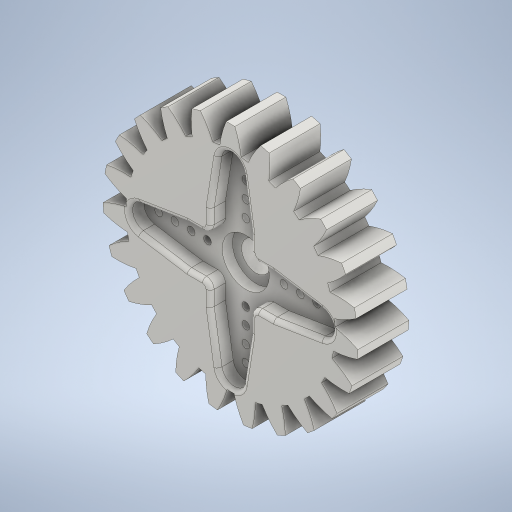
# Autodesk Inventor part: Engrenagem menor
Saved by Autodesk Inventor 2024.1 (Build 281209000, 209)
## iProperties
CustomPartVersion: 1
Created: 2024-11-07
Part Number: Engrenagem menor
Material: Steel
Document SubType Name: Modeling
Designer: dimit
Categories: <?xml version="1.0" encoding="UTF-16"?> <MemberInstance><Categories><FamilyTemplate><FamilyTemplateParameter ValueType="xs:double" Id="1" ObjectReferenceKey="da_z" ObjectType="kUserParameterObject"/><FamilyTemplateParameter ValueType="xs:double" Id="2" ObjectReferenceKey="da_b" ObjectType="kUserParameterObject"/><FamilyTemplateParameter ValueType="xs:double" Id="3" ObjectReferenceKey="da_beta" ObjectType="kUserParameterObject"/><FamilyTemplateParameter ValueType="xs:double" Id="4" ObjectReferenceKey="da_da" ObjectType="kUserParameterObject"/><FamilyTemplateParameter ValueType="xs:double" Id="5" ObjectReferenceKey="da_aw" ObjectType="kUserParameterObject"/><FamilyTemplateParameter ValueType="xs:string" Id="6" ObjectReferenceKey="EAIAABAAAACIAQAAAAAAAIAAAAAAAAAA" ObjectType="83910656" SubObjectId="SurfaceGeometry"/></FamilyTemplate><ParamToTemplateMap><ParamToTemplate CategoryParameter="//CategoryParameter[@InternalName='046C89C9-8512-4d59-83FE-43B91F4F132A']" TemplateParameter="1"/><ParamToTemplate CategoryParameter="//CategoryParameter[@InternalName='2552DF32-E462-4b46-AEBF-C6C7768E72AC']" TemplateParameter="2"/><ParamToTemplate CategoryParameter="//CategoryParameter[@InternalName='C9EE641D-15FC-4fae-A226-E94C4372FDD7']" TemplateParameter="3"/><ParamToTemplate><ParamToTemplate CategoryParameter="//CategoryParameter[@InternalName='00B6519A-459B-49c7-AD84-2E56D39A5744']" ConstantValue="0.000000"/></ParamToTemplate><ParamToTemplate><ParamToTemplate CategoryParameter="//CategoryParameter[@InternalName='04B31F0E-C7A6-4894-AA32-9629BEFACF47']" ConstantValue="1.000000"/></ParamToTemplate><ParamToTemplate><ParamToTemplate CategoryParameter="//CategoryParameter[@InternalName='43CBEC2E-7847-49e7-A936-2F7889FCB2D9']" ConstantValue="0.250000"/></ParamToTemplate><ParamToTemplate><ParamToTemplate CategoryParameter="//CategoryParameter[@InternalName='B1EFC894-105D-4ebd-86BF-FA20ED196853']" ConstantValue="0.333500"/></ParamToTemplate><ParamToTemplate><ParamToTemplate CategoryParameter="//CategoryParameter[@InternalName='51175063-3D10-4879-93E8-6246FE8B403D']" ConstantValue="2060000000.000000"/></ParamToTemplate><ParamToTemplate><ParamToTemplate CategoryParameter="//CategoryParameter[@InternalName='A3A52E27-4454-46a9-B0BD-C932399B70AF']" ConstantValue="0.300000"/></ParamToTemplate><ParamToTemplate><ParamToTemplate CategoryParameter="//CategoryParameter[@InternalName='91B76062-C214-41d9-B1B9-14D2AB99603D']" ConstantValue="0.200000"/></ParamToTemplate><ParamToTemplate><ParamToTemplate CategoryParameter="//CategoryParameter[@InternalName='374E806E-8B8A-4dda-A9AA-1039D6500AD2']" ConstantValue="5.000000"/></ParamToTemplate><ParamToTemplate><ParamToTemplate CategoryParameter="//CategoryParameter[@InternalName='2D373A89-B862-43d6-8D0B-0CBF12AB9F6C']" ConstantValue="0.349066"/></ParamToTemplate><ParamToTemplate CategoryParameter="//CategoryParameter[@InternalName='37777632-D6A2-4fac-9D53-DB8ACD95C989']" TemplateParameter="4"/><ParamToTemplate CategoryParameter="//CategoryParameter[@InternalName='FD1017F1-B727-4f7e-9707-0F86F1FF9423']" TemplateParameter="5"/><ParamToTemplate><ParamToTemplate CategoryParameter="//CategoryParameter[@InternalName='9E1B4470-B2D3-4ff1-B813-535BB4CDF51A']" ConstantValue="3520000.000000"/></ParamToTemplate><ParamToTemplate><ParamToTemplate CategoryParameter="//CategoryParameter[@InternalName='F8452263-BFF6-458c-9FB1-07C4B99E95CD']" ConstantValue="11400000.000000"/></ParamToTemplate><ParamToTemplate><ParamToTemplate CategoryParameter="//CategoryParameter[@InternalName='3E3BB259-FD49-497f-8171-6EBC954A3479']" ConstantValue="2.000000"/></ParamToTemplate><ParamToTemplate CategoryParameter="//CategoryParameter[@InternalName='27C3BAF2-7550-4e4b-AE2C-0DB134B7D9B7']" TemplateParameter="6"/></ParamToTemplateMap><Category DisplayName="Gear" InternalName="DC85795E-93AB-48d5-8EEE-5A27447B64BD" Mnemonic="Gear"><CategoryParameter DisplayName="z" InternalName="046C89C9-8512-4d59-83FE-43B91F4F132A" Mnemonic="z"/><CategoryParameter DisplayName="b" InternalName="2552DF32-E462-4b46-AEBF-C6C7768E72AC" Mnemonic="b"/><CategoryParameter DisplayName="||b|" InternalName="C9EE641D-15FC-4fae-A226-E94C4372FDD7" Mnemonic="beta"/><CategoryParameter DisplayName="x" InternalName="00B6519A-459B-49c7-AD84-2E56D39A5744" Mnemonic="x"/><CategoryParameter DisplayName="a*" InternalName="04B31F0E-C7A6-4894-AA32-9629BEFACF47" Mnemonic="a"/><CategoryParameter DisplayName="c*" InternalName="43CBEC2E-7847-49e7-A936-2F7889FCB2D9" Mnemonic="c"/><CategoryParameter DisplayName="r|.f|*" InternalName="B1EFC894-105D-4ebd-86BF-FA20ED196853" Mnemonic="rf"/><CategoryParameter DisplayName="E" InternalName="51175063-3D10-4879-93E8-6246FE8B403D" Mnemonic="E"/><CategoryParameter DisplayName="||m|" InternalName="A3A52E27-4454-46a9-B0BD-C932399B70AF" Mnemonic="mi"/><Category DisplayName="SpurGear" InternalName="26C5A22E-A91E-4dfd-A3B3-23CCAFAE1764" Mnemonic="SpurGear"><CategoryParameter DisplayName="m" InternalName="91B76062-C214-41d9-B1B9-14D2AB99603D" Mnemonic="m"/><CategoryParameter DisplayName="P" InternalName="374E806E-8B8A-4dda-A9AA-1039D6500AD2" Mnemonic="PP"/><CategoryParameter DisplayName="||a|" InternalName="2D373A89-B862-43d6-8D0B-0CBF12AB9F6C" Mnemonic="alpha"/><CategoryParameter DisplayName="d|.a|" InternalName="37777632-D6A2-4fac-9D53-DB8ACD95C989" Mnemonic="da"/><CategoryParameter DisplayName="a|.w|" InternalName="FD1017F1-B727-4f7e-9707-0F86F1FF9423" Mnemonic="aw"/><CategoryParameter DisplayName="||s||.Flim|" InternalName="9E1B4470-B2D3-4ff1-B813-535BB4CDF51A" Mnemonic="sFlim"/><CategoryParameter DisplayName="||s||.Hlim|" InternalName="F8452263-BFF6-458c-9FB1-07C4B99E95CD" Mnemonic="sHlim"/><CategoryParameter DisplayName="tipo" InternalName="3E3BB259-FD49-497f-8171-6EBC954A3479" Mnemonic="type"/><CategoryParameter DisplayName="PitchDiameter" InternalName="27C3BAF2-7550-4e4b-AE2C-0DB134B7D9B7" Mnemonic="IDS_PITCHDIAM"/></Category></Category></Categories></MemberInstance>
Density: 1 g/cm^3
Appearance: Steel
Author: dimit
Autodesk Inventor part; units mm, degrees
sketch "Sketch1" plane through (0, 0, 0) normal (0, 0, 1) x (1, 0, 0)
  circle A0 centre (0, 0) radius 25
  dimension "d0" = 50
  constraints: 1 centre point
  measures "d0" diameter of A0
extrude "Extrusion1" add sketch "Sketch1" along normal blind 10
ref_plane "Work Plane2" through (0, 0, 5) normal (0, 0, 1) x (1, 0, 0)
sketch "Sketch2" plane through (0, 0, 0) normal (0, 0, -1) x (-1, 0, 0)
  circle A0 centre (0, 0) radius 25 projected
  circle A1 centre (0, 0) radius 23
  dimension "d3" = 46
  constraints: 1 centre point, 1 coincident
  measures "d3" diameter of A1
surface extrude "Diâmetro do flanco" sketch "Sketch2" against normal through all shown no curves A1
ref_plane "Work Plane8" through (0, 0, 0) normal (0.9906859, 0.1361666, 0) x (0, 0, 1)
ref_plane "Work Plane9" through (0, 0, 0) normal (1, 0, 0) x (0, 1, 0)
spur gear teeth "Engrenagem reta" teeth 23 pitch diameter 46 tip diameter 50 root diameter 41 face width 10 start plane through (0, 0, 0) normal (0, 0, -1) x (-1, 0, 0)
sketch "Esboço3" plane through (0, 0, 10) normal (0, 0, 1) x (1, 0, 0)
  circle A0 centre (0, 7.5) radius 0.75
  arc A1 (-5.5, 4) -> (-4, 5.5) centre (-5.5, 5.5) ccw
  line L0 (-4, 5.5) -> (-4, 8.4192)
  line L1 (-4, 5.5) -> (-4, 8.4192)
  arc A2 (-5.5, 4) -> (-4, 5.5) centre (-5.5, 5.5) ccw
  arc A3 (-2.468, -17.8989) -> (2.468, -17.8989) centre (0, -17.5) ccw
  arc A4 (-2.468, -17.8989) -> (2.468, -17.8989) centre (0, -17.5) ccw
  circle A5 centre (10.7, 0) radius 0.75
  line L2 (8.4192, -4) -> (17.8989, -2.468)
  line L3 (17.8989, -2.468) -> (8.4192, -4)
  line L4 (8.4192, 4) -> (17.8989, 2.468)
  line L5 (8.4192, 4) -> (17.8989, 2.468)
  circle A6 centre (13.9, 0) radius 0.75
  circle A7 centre (17.1, 0) radius 0.75
  arc A8 (17.8989, -2.468) -> (17.8989, 2.468) centre (17.5, 0) ccw
  arc A9 (17.8989, -2.468) -> (17.8989, 2.468) centre (17.5, 0) ccw
  arc A10 (5.5, -4) -> (4, -5.5) centre (5.5, -5.5) ccw
  circle A11 centre (7.5, 0) radius 0.75
  line L6 (5.5, 4) -> (8.4192, 4)
  line L7 (5.5, 4) -> (8.4192, 4)
  line L8 (5.5, -4) -> (8.4192, -4)
  line L9 (8.4192, -4) -> (5.5, -4)
  line L10 (4.5575, 0.5) -> (4.5575, -0.5)
  line L11 (3.5904, 0.5) -> (4.5575, 0.5)
  line L12 (4.5575, -0.5) -> (3.5904, -0.5)
  arc A12 (5.5, -4) -> (4, -5.5) centre (5.5, -5.5) ccw
  arc A13 (2.8923, -2.1852) -> (3.5904, -0.5) centre (0, 0) ccw
  arc A14 (3.5904, 0.5) -> (2.8923, 2.1852) centre (0, 0) ccw
  line L13 (3.5762, 2.8691) -> (2.8923, 2.1852)
  line L14 (2.8691, 3.5762) -> (3.5762, 2.8691)
  line L15 (2.1852, 2.8923) -> (2.8691, 3.5762)
  arc A15 (2.1852, 2.8923) -> (0.5, 3.5904) centre (0, 0) ccw
  line L16 (4, 8.4192) -> (2.468, 17.8989)
  arc A16 (2.468, 17.8989) -> (-2.468, 17.8989) centre (0, 17.5) ccw
  line L17 (-4, 8.4192) -> (-2.468, 17.8989)
  circle A17 centre (0, 13.9) radius 0.75
  line L18 (-4, 8.4192) -> (-2.468, 17.8989)
  circle A18 centre (0, 17.1) radius 0.75
  line L19 (2.468, 17.8989) -> (4, 8.4192)
  arc A19 (2.468, 17.8989) -> (-2.468, 17.8989) centre (0, 17.5) ccw
  circle A20 centre (0, 10.7) radius 0.75
  line L20 (-3.5762, 2.8691) -> (-2.8691, 3.5762)
  line L21 (-2.8691, 3.5762) -> (-2.1852, 2.8923)
  line L22 (-2.8923, 2.1852) -> (-3.5762, 2.8691)
  line L23 (-0.5, 3.5904) -> (-0.5, 4.5575)
  line L24 (-0.5, 4.5575) -> (0.5, 4.5575)
  line L25 (0.5, 4.5575) -> (0.5, 3.5904)
  line L26 (-4.5575, 0.5) -> (-3.5904, 0.5)
  arc A21 (-2.8923, 2.1852) -> (-3.5904, 0.5) centre (0, 0) ccw
  line L27 (-4.5575, -0.5) -> (-4.5575, 0.5)
  line L28 (-3.5904, -0.5) -> (-4.5575, -0.5)
  arc A22 (-0.5, 3.5904) -> (-2.1852, 2.8923) centre (0, 0) ccw
  line L29 (4, 5.5) -> (4, 8.4192)
  arc A23 (4, 5.5) -> (5.5, 4) centre (5.5, 5.5) ccw
  arc A24 (4, 5.5) -> (5.5, 4) centre (5.5, 5.5) ccw
  line L30 (4, 8.4192) -> (4, 5.5)
  circle A25 centre (0, 0) radius 2.85
  circle A26 centre (0, 0) radius 4.625
  line L31 (2.8691, -3.5762) -> (2.1852, -2.8923)
  arc A27 (0.5, -3.5904) -> (2.1852, -2.8923) centre (0, 0) ccw
  line L32 (-2.1852, -2.8923) -> (-2.8691, -3.5762)
  arc A28 (-2.1852, -2.8923) -> (-0.5, -3.5904) centre (0, 0) ccw
  line L33 (-0.5, -4.5575) -> (-0.5, -3.5904)
  line L34 (0.5, -4.5575) -> (-0.5, -4.5575)
  line L35 (0.5, -3.5904) -> (0.5, -4.5575)
  line L36 (3.5762, -2.8691) -> (2.8691, -3.5762)
  line L37 (2.8923, -2.1852) -> (3.5762, -2.8691)
  circle A29 centre (0, -17.1) radius 0.75
  circle A30 centre (0, -13.9) radius 0.75
  circle A31 centre (0, -10.7) radius 0.75
  line L38 (-4, -8.4192) -> (-2.468, -17.8989)
  line L39 (-2.468, -17.8989) -> (-4, -8.4192)
  arc A32 (-4, -5.5) -> (-5.5, -4) centre (-5.5, -5.5) ccw
  arc A33 (-4, -5.5) -> (-5.5, -4) centre (-5.5, -5.5) ccw
  arc A34 (-3.5904, -0.5) -> (-2.8923, -2.1852) centre (0, 0) ccw
  line L40 (-3.5762, -2.8691) -> (-2.8923, -2.1852)
  line L41 (-2.8691, -3.5762) -> (-3.5762, -2.8691)
  line L42 (-4, -5.5) -> (-4, -8.4192)
  line L43 (-4, -8.4192) -> (-4, -5.5)
  circle A35 centre (0, -7.5) radius 0.75
  line L44 (4, -5.5) -> (4, -8.4192)
  line L45 (4, -5.5) -> (4, -8.4192)
  line L46 (4, -8.4192) -> (2.468, -17.8989)
  line L47 (4, -8.4192) -> (2.468, -17.8989)
  line L48 (-5.5, 4) -> (-8.4192, 4)
  line L49 (-8.4192, 4) -> (-17.8989, 2.468)
  arc A36 (-17.8989, 2.468) -> (-17.8989, -2.468) centre (-17.5, 0) ccw
  line L50 (-8.4192, -4) -> (-17.8989, -2.468)
  line L51 (-5.5, -4) -> (-8.4192, -4)
  line L52 (-5.5, -4) -> (-8.4192, -4)
  line L53 (-8.4192, -4) -> (-17.8989, -2.468)
  arc A37 (-17.8989, 2.468) -> (-17.8989, -2.468) centre (-17.5, 0) ccw
  line L54 (-17.8989, 2.468) -> (-8.4192, 4)
  line L55 (-8.4192, 4) -> (-5.5, 4)
  circle A38 centre (-7.5, 0) radius 0.75
  circle A39 centre (-10.7, 0) radius 0.75
  circle A40 centre (-13.9, 0) radius 0.75
  circle A41 centre (-17.1, 0) radius 0.75
  point P0 (-20.3157, -17.3312)
  point P1 (0, 0)
  constraints: 112 end point, 48 point on circle, 42 centre point
extrude "Extrusão2" cut sketch "Esboço3" against normal blind 3 contours A1 L0 L17 A16 L16 L29 A23 L6 L4 A8 L2 L8 A10 L44 L46 A3 L38 L42 A32 L51 L50 A36 L49 L48
sketch "Esboço4" plane through (0, 0, 10) normal (0, 0, 1) x (1, 0, 0)
  circle A0 centre (0, 7.5) radius 0.75
  arc A1 (-5.5, 4) -> (-4, 5.5) centre (-5.5, 5.5) ccw
  line L0 (-4, 5.5) -> (-4, 8.4192)
  line L1 (-4, 5.5) -> (-4, 8.4192)
  arc A2 (-5.5, 4) -> (-4, 5.5) centre (-5.5, 5.5) ccw
  arc A3 (-2.468, -17.8989) -> (2.468, -17.8989) centre (0, -17.5) ccw
  arc A4 (-2.468, -17.8989) -> (2.468, -17.8989) centre (0, -17.5) ccw
  circle A5 centre (10.7, 0) radius 0.75
  line L2 (8.4192, -4) -> (17.8989, -2.468)
  line L3 (17.8989, -2.468) -> (8.4192, -4)
  line L4 (8.4192, 4) -> (17.8989, 2.468)
  line L5 (8.4192, 4) -> (17.8989, 2.468)
  circle A6 centre (13.9, 0) radius 0.75
  circle A7 centre (17.1, 0) radius 0.75
  arc A8 (17.8989, -2.468) -> (17.8989, 2.468) centre (17.5, 0) ccw
  arc A9 (17.8989, -2.468) -> (17.8989, 2.468) centre (17.5, 0) ccw
  arc A10 (5.5, -4) -> (4, -5.5) centre (5.5, -5.5) ccw
  circle A11 centre (7.5, 0) radius 0.75
  line L6 (5.5, 4) -> (8.4192, 4)
  line L7 (5.5, 4) -> (8.4192, 4)
  line L8 (5.5, -4) -> (8.4192, -4)
  line L9 (8.4192, -4) -> (5.5, -4)
  line L10 (4.5575, 0.5) -> (4.5575, -0.5)
  line L11 (3.5904, 0.5) -> (4.5575, 0.5)
  line L12 (4.5575, -0.5) -> (3.5904, -0.5)
  arc A12 (5.5, -4) -> (4, -5.5) centre (5.5, -5.5) ccw
  arc A13 (2.8923, -2.1852) -> (3.5904, -0.5) centre (0, 0) ccw
  arc A14 (3.5904, 0.5) -> (2.8923, 2.1852) centre (0, 0) ccw
  line L13 (3.5762, 2.8691) -> (2.8923, 2.1852)
  line L14 (2.8691, 3.5762) -> (3.5762, 2.8691)
  line L15 (2.1852, 2.8923) -> (2.8691, 3.5762)
  arc A15 (2.1852, 2.8923) -> (0.5, 3.5904) centre (0, 0) ccw
  line L16 (4, 8.4192) -> (2.468, 17.8989)
  arc A16 (2.468, 17.8989) -> (-2.468, 17.8989) centre (0, 17.5) ccw
  line L17 (-4, 8.4192) -> (-2.468, 17.8989)
  circle A17 centre (0, 13.9) radius 0.75
  line L18 (-4, 8.4192) -> (-2.468, 17.8989)
  circle A18 centre (0, 17.1) radius 0.75
  line L19 (2.468, 17.8989) -> (4, 8.4192)
  arc A19 (2.468, 17.8989) -> (-2.468, 17.8989) centre (0, 17.5) ccw
  circle A20 centre (0, 10.7) radius 0.75
  line L20 (-3.5762, 2.8691) -> (-2.8691, 3.5762)
  line L21 (-2.8691, 3.5762) -> (-2.1852, 2.8923)
  line L22 (-2.8923, 2.1852) -> (-3.5762, 2.8691)
  line L23 (-0.5, 3.5904) -> (-0.5, 4.5575)
  line L24 (-0.5, 4.5575) -> (0.5, 4.5575)
  line L25 (0.5, 4.5575) -> (0.5, 3.5904)
  line L26 (-4.5575, 0.5) -> (-3.5904, 0.5)
  arc A21 (-2.8923, 2.1852) -> (-3.5904, 0.5) centre (0, 0) ccw
  line L27 (-4.5575, -0.5) -> (-4.5575, 0.5)
  line L28 (-3.5904, -0.5) -> (-4.5575, -0.5)
  arc A22 (-0.5, 3.5904) -> (-2.1852, 2.8923) centre (0, 0) ccw
  line L29 (4, 5.5) -> (4, 8.4192)
  arc A23 (4, 5.5) -> (5.5, 4) centre (5.5, 5.5) ccw
  arc A24 (4, 5.5) -> (5.5, 4) centre (5.5, 5.5) ccw
  line L30 (4, 8.4192) -> (4, 5.5)
  circle A25 centre (0, 0) radius 2.85
  circle A26 centre (0, 0) radius 4.625
  line L31 (2.8691, -3.5762) -> (2.1852, -2.8923)
  arc A27 (0.5, -3.5904) -> (2.1852, -2.8923) centre (0, 0) ccw
  line L32 (-2.1852, -2.8923) -> (-2.8691, -3.5762)
  arc A28 (-2.1852, -2.8923) -> (-0.5, -3.5904) centre (0, 0) ccw
  line L33 (-0.5, -4.5575) -> (-0.5, -3.5904)
  line L34 (0.5, -4.5575) -> (-0.5, -4.5575)
  line L35 (0.5, -3.5904) -> (0.5, -4.5575)
  line L36 (3.5762, -2.8691) -> (2.8691, -3.5762)
  line L37 (2.8923, -2.1852) -> (3.5762, -2.8691)
  circle A29 centre (0, -17.1) radius 0.75
  circle A30 centre (0, -13.9) radius 0.75
  circle A31 centre (0, -10.7) radius 0.75
  line L38 (-4, -8.4192) -> (-2.468, -17.8989)
  line L39 (-2.468, -17.8989) -> (-4, -8.4192)
  arc A32 (-4, -5.5) -> (-5.5, -4) centre (-5.5, -5.5) ccw
  arc A33 (-4, -5.5) -> (-5.5, -4) centre (-5.5, -5.5) ccw
  arc A34 (-3.5904, -0.5) -> (-2.8923, -2.1852) centre (0, 0) ccw
  line L40 (-3.5762, -2.8691) -> (-2.8923, -2.1852)
  line L41 (-2.8691, -3.5762) -> (-3.5762, -2.8691)
  line L42 (-4, -5.5) -> (-4, -8.4192)
  line L43 (-4, -8.4192) -> (-4, -5.5)
  circle A35 centre (0, -7.5) radius 0.75
  line L44 (4, -5.5) -> (4, -8.4192)
  line L45 (4, -5.5) -> (4, -8.4192)
  line L46 (4, -8.4192) -> (2.468, -17.8989)
  line L47 (4, -8.4192) -> (2.468, -17.8989)
  line L48 (-5.5, 4) -> (-8.4192, 4)
  line L49 (-8.4192, 4) -> (-17.8989, 2.468)
  arc A36 (-17.8989, 2.468) -> (-17.8989, -2.468) centre (-17.5, 0) ccw
  line L50 (-8.4192, -4) -> (-17.8989, -2.468)
  line L51 (-5.5, -4) -> (-8.4192, -4)
  line L52 (-5.5, -4) -> (-8.4192, -4)
  line L53 (-8.4192, -4) -> (-17.8989, -2.468)
  arc A37 (-17.8989, 2.468) -> (-17.8989, -2.468) centre (-17.5, 0) ccw
  line L54 (-17.8989, 2.468) -> (-8.4192, 4)
  line L55 (-8.4192, 4) -> (-5.5, 4)
  circle A38 centre (-7.5, 0) radius 0.75
  circle A39 centre (-10.7, 0) radius 0.75
  circle A40 centre (-13.9, 0) radius 0.75
  circle A41 centre (-17.1, 0) radius 0.75
  point P0 (0, 0)
  point P1 (0, 0)
  constraints: 112 end point, 48 point on circle, 42 centre point
extrude "Extrusão3" cut sketch "Esboço4" against normal blind 10 contours A0 | A5 | A6 | A7 | A11 | A17 | A18 | A20 | A25 | A29 | A30 | A31 | A35 | A38 | A39 | A40 | A41
sketch "Esboço5" plane through (0, 0, 10) normal (0, 0, 1) x (1, 0, 0)
  circle A0 centre (0, 0) radius 4.625
  circle A1 centre (0, 0) radius 2.85
  constraints: 2 centre point, 2 coincident
extrude "Extrusão4" cut sketch "Esboço5" against normal blind 5
fillet "Arredondamento1" radius 0.8 24 edges at (0, -20, 10) (3.234, -13.159, 10) (-3.234, -13.159, 10) (-20, 0, 10) (-13.159, 3.234, 10) (-13.159, -3.234, 10) (-6.9596, -4, 10) (-4, -6.9596, 10) (-4.4393, -4.4393, 10) (4.4393, -4.4393, 10) (6.9596, -4, 10) (4, -6.9596, 10) (20, 0, 10) (13.159, 3.234, 10) (13.159, -3.234, 10) (4.4393, 4.4393, 10) (4, 6.9596, 10) (6.9596, 4, 10) (0, 20, 10) (-3.234, 13.159, 10) (3.234, 13.159, 10) (-4.4393, 4.4393, 10) (-6.9596, 4, 10) (-4, 6.9596, 10)
equation "\"d0\" = da_da"
equation "\"d1\" = da_b"
equation "\"d3\" = da_d"
equation "\"da_da\" = 50"
equation "\"da_b\" = 10"
equation "\"da_d\" = 46"
body "Solid1"
body "Srf1"
